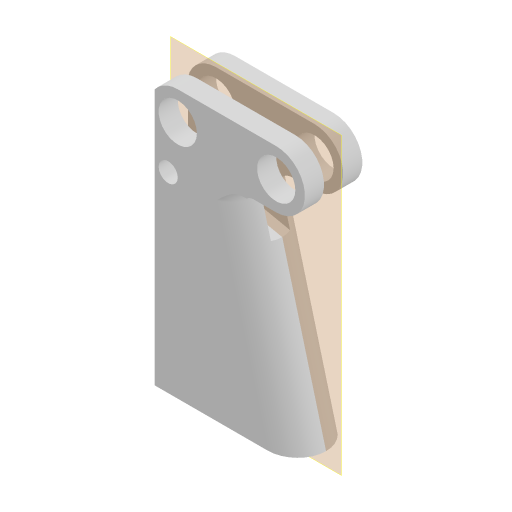
# Autodesk Inventor part: wedge
Saved by Autodesk Inventor 2023 (Build 270158000, 158)
## iProperties
Created: 2022-10-23
Part Number: wedge
Material: Generic
Document SubType Name: Modeling
Designer: deli
Density: 1 g/cm^3
Appearance: Default
Author: deli
Autodesk Inventor part; units mm, degrees
ref_plane "YZ Plane" through (0, 0, 0) normal (1, 0, 0) x (0, 1, 0)
ref_plane "XZ Plane" through (0, 0, 0) normal (0, 1, 0) x (-1, 0, 0)
ref_plane "XY Plane" through (0, 0, 0) normal (0, 0, 1) x (1, 0, 0)
sketch "Sketch1" plane through (0, 0, 0) normal (0, 0, 1) x (1, 0, 0)
  line L0 (-11.177, 7.2143) -> (-11.177, -42.7857)
  line L1 (-11.177, -42.7857) -> (19.823, -42.7857)
  line L2 (19.823, -42.7857) -> (8.7078, -1.3034)
  line L3 (15.397, 13.2143) -> (-5.177, 13.2143)
  circle A0 centre (-7.177, -2.7857) radius 2
  line L4 (-11.177, -42.7857) -> (-11.177, -2.7857) construction
  line L5 (-11.177, -46.7857) -> (-3.177, -46.7857) construction
  line L6 (-3.177, -46.7857) -> (-3.177, -2.7857) construction
  arc A1 (-3.177, -2.7857) -> (-11.177, -2.7857) centre (-7.177, -2.7857) ccw construction
  line L7 (-12.3103, -19.3446) -> (19.4397, -19.3446) construction
  line L8 (3.5647, -19.3446) -> (3.5647, -41.2883) construction
  line L9 (19.4397, -19.3446) -> (19.8228, -41.2883) construction
  line L10 (-17.3867, -4.7049) -> (25.318, -13.7821) construction
  circle A2 centre (24.2015, -19.2615) radius 4.7625 construction
  circle A3 centre (21.3465, -41.2617) radius 1.524 construction
  line L11 (-12.6933, -41.2883) -> (19.8228, -41.2883) construction
  circle A4 centre (-14.2171, -41.2617) radius 1.524 construction
  line L12 (-12.3103, -19.3446) -> (-12.6933, -41.2883) construction
  line L13 (-11.177, -42.7857) -> (-15.177, -42.7857) construction
  line L14 (-15.177, -42.7857) -> (-11.177, -46.7857) construction
  circle A5 centre (-14.2171, -41.2617) radius 40.1639 construction
  circle A6 centre (-5.177, 7.2143) radius 4
  circle A7 centre (15.397, 7.2143) radius 4
  line L15 (21.397, 7.2143) -> (21.397, 7.2143)
  line L16 (15.397, 1.2143) -> (10.6397, 1.2143)
  arc A8 (10.6397, 1.2143) -> (8.7078, -1.3034) centre (10.6397, -0.7857) ccw
  arc A9 (-5.177, 13.2143) -> (-11.177, 7.2143) centre (-5.177, 7.2143) ccw
  arc A10 (21.397, 7.2143) -> (15.397, 13.2143) centre (15.397, 7.2143) ccw
  arc A11 (15.397, 1.2143) -> (21.397, 7.2143) centre (15.397, 7.2143) ccw
  point P0 (0, 0)
  point P1 (-11.177, 13.2143)
  point P2 (21.397, 13.2143)
  point P3 (8.0332, 1.2143)
  dimension "d52" = 9.525
  dimension "d53" = 3.048
  dimension "d0" = 31
  dimension "d1" = 4
  dimension "d4" = 4
  dimension "d5" = 16
  dimension "d7" = 8
  dimension "d8" = 40
  dimension "d9" = 44
  dimension "d11" = 31.75
  dimension "d13" = 21.9437
  dimension "d54" = 32.5161
  dimension "d56" = 4
  dimension "d58" = 4
  dimension "d60" = 35.5636
  dimension "d61" = 3.0401
  dimension "d63" = 75
  dimension "d64" = 0
  dimension "d66" = 78
  dimension "d69" = 8
  dimension "d70" = 8
  dimension "d71" = 20.574
  dimension "d72" = 6
  dimension "d73" = 6
  dimension "d74" = 6
  dimension "d75" = 6
  dimension "d76" = 2
  dimension "d77" = 6
  dimension "d78" = 6
  constraints: 34 end point, 11 tangent, 10 point on circle, 8 centre point, 7 point on line, 5 perpendicular, 3 vertical, 2 horizontal, 2 midpoint, 2 parallel, 1 coincident, 1 concentric, 1 equal radius, 15 other
  measures "d0" distance of L0.end L1.end
  measures "d1" diameter of A0
  measures "d4" distance from line of L0 A0.centre
  measures "d5" distance from line of L3 A0.centre
  measures "d7" distance between parallel lines of L6 L4
  measures "d8" distance from line of L1 A0.centre
  measures "d9" distance of L5.end L6.end
  measures "d11" distance of L7.end L7.start
  measures "d13" distance of L8.end L8.start
  measures "d54" distance of L9.end L11.start
  measures "d56" distance of L4.start L13.end
  measures "d58" distance between parallel lines of L5 L13
  measures "d60" distance of point (21.347, -41.262) point (-14.217, -41.262)
  measures "d61" horizontal distance of L0.end point (-14.217, -41.262)
  measures "d63" angle of L2 L1
  measures "d64" distance from line of L0 L4.start
  measures "d66" angle of L6 L10
  measures "d69" diameter of A6
  measures "d70" diameter of A7
  measures "d71" distance of A7.centre A6.centre
  measures "d72" distance from line of L0 A6.centre
  measures "d73" distance from line of L3 A6.centre
  measures "d74" distance from line of L3 A7.centre
  measures "d75" distance from line of L15 A7.centre
  measures "d76" radius of A8
  measures "d77" radius of A9
  measures "d78" radius of A11
extrude "Extrusion1" add sketch "Sketch1" along normal blind 4
sketch "Sketch2" plane through (0, 0, 4) normal (0, 0, 1) x (1, 0, 0)
  line L0 (15.397, 13.2143) -> (-5.177, 13.2143) projected
  line L1 (-7.0087, 13.2143) -> (7.257, -44.5429)
  line L2 (19.823, -42.7857) -> (8.7078, -1.3034) projected
  circle A0 centre (-7.177, -2.7857) radius 2 projected
  line L3 (-9.7939, -8.8719) -> (-1.4688, -42.5779) construction
  line L4 (-1.4688, -42.5779) -> (-11.177, -44.9758) construction
  line L5 (-11.177, -44.9758) -> (-10.2178, -48.8591) construction
  line L6 (-10.2178, -48.8591) -> (7.257, -44.5429) construction
  line L7 (-11.177, 7.2143) -> (-11.177, -42.7857) construction
  line L8 (-11.177, -42.7857) -> (19.823, -42.7857) projected
  line L9 (-11.177, -6.9187) -> (10.0266, -6.2249)
  line L10 (-11.177, -3.9802) -> (10.6693, -8.6238)
  line L11 (-9.9165, 3.9306) -> (8.3455, 0.0489)
  line L12 (-10.5708, -0.8957) -> (8.432, -0.2739)
  point P0 (0, 0)
  point P1 (8.0332, 13.2143)
  point P2 (-11.177, 13.2143)
  point P3 (6.823, -42.7857)
  point P4 (-3.5801, -0.667)
  point P5 (-2.2955, -5.868)
  point P6 (8.0332, 1.2143)
  point P7 (8.7078, -1.3034)
  dimension "d22" = 4
  dimension "d23" = 8
  dimension "d24" = 4
  dimension "d25" = 10
  dimension "d26" = 40
  dimension "d31" = 4
  dimension "d32" = 78
  dimension "d33" = 2
  dimension "d34" = 78
  dimension "d35" = 2
  dimension "d36" = 6
  constraints: 18 end point, 5 parallel, 4 point on line, 1 perpendicular, 5 other
  measures "d22" distance from line of L1 A0.centre
  measures "d23" distance between parallel lines of L1 L3
  measures "d24" distance between parallel lines of L6 L4
  measures "d25" distance of L3.end L4.end
  measures "d26" distance from line of L4 A0.centre
  measures "d31" distance from line of A0.centre L9
  measures "d32" angle of L9 L1
  measures "d33" distance from line of A0.centre L10
  measures "d34" angle of L7 L10
  measures "d35" distance from line of L12 A0.centre
  measures "d36" distance from line of A0.centre L11
extrude "Extrusion2" add sketch "Sketch2" along normal blind 4 contours L10 L9 L1 | L9 L10 L2 L8 L1
sketch "Sketch3" plane through (0, 0, 8) normal (0, 0, 1) x (1, 0, 0)
  line L0 (-11.177, -42.7857) -> (19.823, -42.7857) projected
  line L1 (-11.177, 7.2143) -> (-11.177, -42.7857) projected
  line L2 (15.397, 13.2143) -> (-5.177, 13.2143) projected
  line L3 (19.823, -42.7857) -> (8.7078, -1.3034) projected
  circle A0 centre (-7.177, -2.7857) radius 2 projected
  arc A1 (15.397, 1.2143) -> (15.397, 13.2143) centre (15.397, 7.2143) ccw projected
  line L4 (10.6397, 1.2143) -> (15.397, 1.2143) projected
  arc A2 (10.6397, 1.2143) -> (8.7078, -1.3034) centre (10.6397, -0.7857) ccw projected
  arc A3 (-5.177, 13.2143) -> (-11.177, 7.2143) centre (-5.177, 7.2143) ccw projected
  circle A4 centre (-5.177, 7.2143) radius 4 projected
  circle A5 centre (15.397, 7.2143) radius 4 projected
  point P0 (0, 0)
extrude "Extrusion3" add sketch "Sketch3" along normal blind 4
sketch "Sketch7" plane through (-11.177, -42.7857, 0) normal (0, -1, 0) x (1, 0, 0)
  circle A0 centre (15.5, 6) radius 15.5
  line L0 (0, 12) -> (31, 12) projected
  ellipse E0 centre (23.2354, 6) end of major axis (15.4709, 6) minor radius 7.5 (27.8942, 0) -> (27.8942, 12) ccw projected
  circle A1 centre (15.5, 6) radius 19.8481
  line L1 (14.8035, 26.6038) -> (14.8035, -21.3363)
  point P0 (11.177, 0)
  point P1 (14.8035, -13.8359)
  point P2 (14.8035, -9.4843)
  point P3 (14.8035, 21.4843)
  point P4 (14.8035, 25.8359)
  dimension "d48" = 31
  dimension "d49" = 6
  constraints: 2 centre point, 2 end point, 1 coincident, 1 vertical, 2 other
  measures "d48" diameter of A0
  measures "d49" distance from line of A0.centre L0
extrude "Extrusion7" cut sketch "Sketch7" against normal blind 60 contours L1 A1 A0 picked at (13.2623, 24.1473)
ref_plane "Work Plane1" through (0, 0, 6) normal (0, 0, 1) x (1, 0, 0)
sketch "Sketch8" plane through (0, 0, 6) normal (0, 0, 1) x (1, 0, 0)
  line L0 (3.1591, -3.7773) -> (16.2709, -52.7113)
  line L1 (19.823, -42.7857) -> (8.7078, -1.3034) projected
  line L2 (10.6397, 1.2143) -> (15.397, 1.2143) projected
  arc A0 (10.6397, 1.2143) -> (8.7078, -1.3034) centre (10.6397, -0.7857) ccw projected
  line L3 (10.6397, 1.2143) -> (15.397, 1.2143) projected
  line L4 (15.397, 1.2143) -> (19.823, -42.7857)
  line L5 (19.823, -42.7857) -> (42.5927, -42.7857)
  line L6 (42.5927, -42.7857) -> (42.5927, 1.2143)
  line L7 (42.5927, 1.2143) -> (15.397, 1.2143)
  arc A1 (15.397, 1.2143) -> (15.397, 13.2143) centre (15.397, 7.2143) ccw projected
  arc A2 (15.397, 1.2143) -> (15.397, 13.2143) centre (15.397, 7.2143) ccw projected
  line L8 (21.397, 7.2143) -> (42.5927, 1.2143)
  point P0 (0, 0)
  dimension "d80" = 6
  constraints: 12 end point, 2 perpendicular, 2 point on circle, 1 parallel, 1 vertical
  measures "d80" distance between parallel lines of L1 L0
revolve "Revolution1" cut sketch "Sketch8" angle 180 mid plane about axis through (3.1591, -3.7773, 6) along (0.258819, -0.9659258, 0) contours L1 A0 L2 L4 | L4 L7 L6 L5
body "Solid1"
